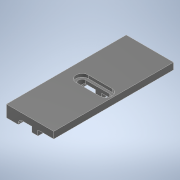
# Autodesk Inventor part: Carrier Clip V1
Saved by Autodesk Inventor 2022 (Build 260153000, 153)
## iProperties
Created: 2022-04-14
Part Number: Carrier Clip V1
Material: Acetal Resin, Black
Document SubType Name: Modeling
Designer: Caleb
Density: 1.425 g/cm^3
Appearance: Smooth - Black
Author: Caleb
Autodesk Inventor part; units mm, degrees
ref_plane "YZ Plane" through (0, 0, 0) normal (1, 0, 0) x (0, 1, 0)
ref_plane "XZ Plane" through (0, 0, 0) normal (0, 1, 0) x (-1, 0, 0)
ref_plane "XY Plane" through (0, 0, 0) normal (0, 0, 1) x (1, 0, 0)
sketch "Sketch1" plane through (0, 0, 0) normal (0, 1, 0) x (-1, 0, 0)
  line L0 (-9.525, -24.13) -> (9.525, -24.13)
  line L1 (9.525, -24.13) -> (9.525, 24.13)
  line L2 (9.525, 24.13) -> (-9.525, 24.13)
  line L3 (-9.525, 24.13) -> (-9.525, -24.13)
  line L4 (-9.525, -24.13) -> (9.525, 24.13) construction
  line L5 (9.525, -24.13) -> (-9.525, 24.13) construction
  point P0 (0, 0)
  dimension "d0" = 19.05
  dimension "d1" = 48.26
  constraints: 12 end point, 2 midpoint, 2 parallel, 1 horizontal, 1 perpendicular
  measures "d0" distance of L2.end L1.end
  measures "d1" distance of L0.end L1.end
extrude "Extrusion1" add sketch "Sketch1" along normal blind 4.7625
sketch "Sketch2" plane through (-9.525, 0, 24.13) normal (0, 0, 1) x (1, 0, 0)
  line L0 (19.05, 0) -> (19.05, 4.7625) projected
  line L1 (19.05, 2.1) -> (6.35, 2.1)
  line L2 (4.7625, 0.5125) -> (4.7625, 0)
  line L3 (0, 0) -> (19.05, 0) projected
  line L4 (0, 4.7625) -> (19.05, 4.7625) projected
  arc A0 (6.35, 2.1) -> (4.7625, 0.5125) centre (6.35, 0.5125) ccw
  point P0 (9.525, 0)
  point P1 (4.7625, 2.1)
  dimension "d4" = 14.2875
  dimension "d6" = 1.5875
  dimension "d21" = 2.1
  constraints: 4 end point, 4 point on line, 2 point on circle, 2 tangent, 1 centre point, 1 perpendicular, 1 vertical
  measures "d4" distance of L1.start point (4.763, 2.1)
  measures "d6" radius of A0
  measures "d21" distance between parallel lines of L3 L1
extrude "Extrusion2" cut sketch "Sketch2" against normal through all
sketch "Sketch3" plane through (-3.175, 2.1, 24.13) normal (0, -1, 0) x (1, 0, 0)
  line L0 (1.4801, -24.13) -> (10.1501, -24.13)
  line L1 (12.7, 0) -> (12.7, -48.26) projected
  circle A0 centre (9.525, -4.33) radius 1.1
  circle A1 centre (9.525, -43.93) radius 1.1
  point P0 (3.175, -24.13)
  dimension "d9" = 39.6
  dimension "d10" = 3.175
  dimension "d11" = 2.2
  dimension "d12" = 2.2
  constraints: 2 centre point, 2 coincident, 2 end point, 1 horizontal, 1 point on line, 1 symmetric about line, 1 vertical alignment
  measures "d9" distance of point (9.525, -4.33) point (9.525, -43.93)
  measures "d10" distance from line of L1 point (9.525, -4.33)
  measures "d11" diameter of A0
  measures "d12" diameter of A1
extrude "Extrusion3" add sketch "Sketch3" along normal blind 1.5875
fillet "Fillet1" radius 0.7937 2 edges at (5.25, 0.5125, 19.8) (5.25, 0.5125, -19.8)
sketch "Sketch6" plane through (-3.175, 2.1, 24.13) normal (0, -1, 0) x (1, 0, 0)
  line L0 (-6.35, 0) -> (12.7, 0) projected
  line L1 (12.7, -48.26) -> (-6.35, -48.26) projected
  line L2 (6.35, 0) -> (3.81, 0)
  line L3 (3.81, 0) -> (3.81, -48.26)
  line L4 (3.81, -48.26) -> (6.35, -48.26)
  line L5 (6.35, -48.26) -> (6.35, 0)
  line L6 (12.7, 0) -> (12.7, -48.26) projected
  point P0 (3.175, -24.13)
  point P1 (3.81, 0)
  dimension "d25" = 6.35
  dimension "d26" = 2.54
  constraints: 8 end point, 2 parallel, 2 point on line, 1 horizontal, 1 perpendicular
  measures "d25" distance between parallel lines of L5 L6
  measures "d26" distance between parallel lines of L3 L5
extrude "Extrusion6" add sketch "Sketch6" along normal up to surface (2.1 mm away) contours L0 L5 L1 L3
sketch "Sketch4" plane through (0, 4.7625, 0) normal (0, 1, 0) x (1, 0, 0)
  line L0 (6.35, 0) -> (-3.175, 0) construction
  line L1 (-3.175, -24.13) -> (-3.175, 24.13) projected
  line L2 (6.35, 1.524) -> (-3.175, 1.524)
  line L3 (-3.175, -1.524) -> (6.35, -1.524)
  arc A0 (6.35, -1.524) -> (6.35, 1.524) centre (6.35, 0) ccw
  arc A1 (-3.175, 1.524) -> (-3.175, -1.524) centre (-3.175, 0) ccw
  line L4 (-9.525, 24.13) -> (-9.525, -24.13) projected
  line L5 (9.525, -24.13) -> (9.525, 24.13) projected
  point P0 (0, 0)
  point P1 (1.5875, 0)
  dimension "d16" = 1.524
  dimension "d17" = 9.525
  dimension "d30" = 3.175
  constraints: 8 end point, 4 point on circle, 4 tangent, 2 centre point, 1 horizontal alignment, 1 midpoint, 1 parallel, 1 perpendicular
  measures "d16" radius of A1
  measures "d17" distance of L3.start L3.end
  measures "d30" distance from line of L5 L0.start
extrude "Extrusion4" cut sketch "Sketch4" against normal through all
sketch "Sketch7" plane through (0, 4.7625, 0) normal (0, 1, 0) x (1, 0, 0)
  line L0 (-5.715, 0) -> (8.89, 0) construction
  line L1 (-3.175, -2.54) -> (6.35, -2.54)
  line L2 (6.35, 2.54) -> (-3.175, 2.54)
  arc A0 (-3.175, 2.54) -> (-3.175, -2.54) centre (-3.175, 0) ccw
  arc A1 (6.35, -2.54) -> (6.35, 2.54) centre (6.35, 0) ccw
  arc A2 (-3.175, 1.524) -> (-3.175, -1.524) centre (-3.175, 0) ccw projected
  arc A3 (6.35, -1.524) -> (6.35, 1.524) centre (6.35, 0) ccw projected
  point P0 (0, 0)
  point P1 (1.5875, 0)
  dimension "d31" = 5.08
  dimension "d32" = 0
  dimension "d33" = 0
  constraints: 8 end point, 6 point on circle, 4 tangent, 2 centre point, 2 point on line, 1 horizontal, 1 midpoint, 1 parallel
  measures "d31" distance between parallel lines of L2 L1
  measures "d32" distance of A0.centre A2.centre
  measures "d33" distance of A1.centre A3.centre
extrude "Extrusion7" cut sketch "Sketch7" against normal blind 1.27
equation "\"d12\" = d11"
body "Solid1"
